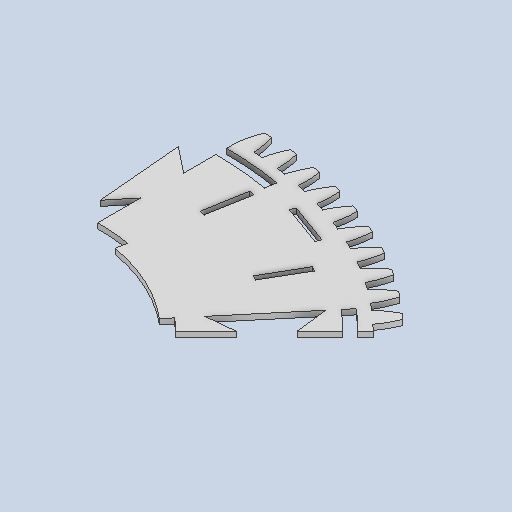
# Autodesk Inventor part: Base Plate Bottom v3
Saved by Autodesk Inventor 2023 (Build 270158000, 158)
## iProperties
Created: 2023-02-13
Part Number: Base Plate Bottom v3
Material: Generic
Document SubType Name: Sheet Metal
Designer: cheng
Density: 1 g/cm^3
Appearance: Default
Sheet Metal Rule: Default
Author: cheng
Autodesk Inventor part; units mm, degrees
(part 1 of 2)
ref_plane "YZ Plane" through (0, 0, 0) normal (1, 0, 0) x (0, 1, 0)
ref_plane "XZ Plane" through (0, 0, 0) normal (0, 1, 0) x (-1, 0, 0)
ref_plane "XY Plane" through (0, 0, 0) normal (0, 0, 1) x (1, 0, 0)
sketch "Sketch2" plane through (0, 0, 0) normal (0, 1, 0) x (-1, 0, 0)
  circle A0 centre (0, 0) radius 325
  circle A1 centre (0, 0) radius 165
  line L0 (0, 0) -> (0, -325)
  line L1 (0, 0) -> (-229.8097, -229.8097)
  line L2 (0, 0) -> (28.3256, -323.7633)
  line L3 (0, 0) -> (-208.906, -248.9644)
  circle A2 centre (0, 0) radius 275 construction
  circle A3 centre (0, 0) radius 195
  circle A4 centre (0, 0) radius 215
  circle A5 centre (0, 0) radius 255 construction
  line L4 (16.9954, -194.258) -> (0, -215)
  line L5 (23.9678, -273.9535) -> (0, -255)
  line L6 (-125.3436, -149.3787) -> (-152.028, -152.028)
  line L7 (-176.7666, -210.6622) -> (-180.3122, -180.3122)
  line L8 (0, 0) -> (-111.1565, -305.4001) construction
  circle A6 centre (0, 0) radius 235 construction
  circle A7 centre (0, 0) radius 275 construction
  line L9 (0, 0) -> (-17.0092, -324.5546) construction
  line L10 (0, 0) -> (-8.5075, -324.8886) construction
  circle A8 centre (0, 0) radius 305
  arc A9 (-5.1732, -324.9588) -> (0, -305) centre (-79.3819, -295.0744) ccw
  arc A10 (-15.9625, -304.582) -> (-11.8409, -324.7842) centre (63.8301, -298.8246) ccw
  arc A11 (20.3387, -324.363) -> (23.93, -304.0598) centre (-55.9859, -300.393) ccw
  arc A12 (7.984, -304.8955) -> (13.6779, -324.712) centre (87.0788, -292.8953) ccw
  arc A13 (45.7252, -321.7673) -> (47.7125, -301.2449) centre (-32.2447, -303.8596) ccw
  arc A14 (31.8812, -303.3292) -> (39.1123, -322.6379) centre (109.7907, -285.1603) ccw
  arc A15 (70.8298, -317.1879) -> (71.2008, -296.5728) centre (-8.3048, -305.4528) ccw
  arc A16 (55.5818, -299.8927) -> (64.3057, -318.5746) centre (131.8257, -275.6672) ccw
  arc A17 (95.4978, -310.6528) -> (94.2502, -290.0722) centre (15.6864, -305.1628) ccw
  arc A18 (78.9398, -294.6074) -> (89.1025, -312.5472) centre (153.0479, -264.4745) ccw
  arc A19 (119.5769, -302.2025) -> (116.7184, -281.7833) centre (39.5808, -302.9913) ccw
  arc A20 (101.8111, -287.5057) -> (113.35, -304.5928) centre (173.3265, -251.6512) ccw
  arc A21 (142.9188, -291.889) -> (138.4671, -271.757) centre (63.2312, -298.9518) ccw
  arc A22 (124.0547, -278.6314) -> (136.8987, -294.7605) centre (192.5365, -237.2764) ccw
  arc A23 (165.3796, -279.776) -> (159.3621, -260.0553) centre (86.4918, -293.0692) ccw
  arc A24 (145.5334, -268.0392) -> (159.6033, -283.1109) centre (210.5595, -221.4387) ccw
  arc A25 (186.8208, -265.938) -> (179.2745, -246.7502) centre (109.2191, -285.3797) ccw
  arc A26 (166.1149, -255.7945) -> (181.3239, -269.7159) centre (227.2843, -204.2358) ccw
  arc A27 (207.1101, -250.4604) -> (198.0817, -231.9238) centre (131.273, -275.9308) ccw
  arc A28 (185.6722, -241.9728) -> (201.9266, -254.6579) centre (242.6078, -185.7736) ccw
  arc A29 (226.1226, -233.4386) -> (215.6676, -215.6676) centre (152.5177, -264.7806) ccw
  arc A30 (204.0848, -226.6592) -> (221.2844, -238.0299) centre (256.4356, -166.1662) ccw
  arc A31 (243.7409, -214.9776) -> (231.9238, -198.0817) centre (172.8219, -251.998) ccw
  arc A32 (221.2392, -209.9481) -> (239.2778, -219.9344) centre (268.6823, -145.5342) ccw
  arc A33 (259.8565, -195.1912) -> (246.7502, -179.2745) centre (192.0607, -237.6617) ccw
  arc A34 (237.0295, -191.9427) -> (255.7961, -200.4829) centre (279.2725, -124.005) ccw
  arc A35 (274.3699, -174.2014) -> (260.0553, -159.3621) centre (210.1154, -221.8601) ccw
  arc A36 (251.3585, -172.7539) -> (270.7372, -179.7953) centre (288.1409, -101.7113) ccw
  arc A37 (287.1918, -152.1376) -> (271.757, -138.4671) centre (226.8746, -204.6908) ccw
  arc A38 (264.1377, -152.5) -> (284.0092, -157.9993) centre (295.2329, -78.7905) ccw
  arc A39 (298.2431, -129.1358) -> (281.7833, -116.7184) centre (242.2351, -186.2594) ccw
  arc A40 (275.2885, -131.3059) -> (295.5302, -135.2291) centre (300.5046, -55.3839) ccw
  arc A41 (307.4556, -105.3378) -> (290.0722, -94.2502) centre (256.1021, -166.6797) ccw
  arc A42 (284.742, -109.3022) -> (305.2291, -111.6252) centre (303.9236, -31.6358) ccw
  arc A43 (314.7725, -80.8904) -> (296.5728, -71.2008) centre (268.3902, -146.0723) ccw
  arc A44 (292.44, -86.6247) -> (313.0462, -87.3331) centre (305.4688, -7.6927) ccw
  arc A45 (320.1488, -55.9443) -> (301.2449, -47.7125) centre (279.0235, -124.5644) ccw
  arc A46 (298.335, -63.4131) -> (318.9333, -62.5025) centre (305.1308, 16.2978) ccw
  arc A47 (323.5512, -30.6533) -> (304.0598, -23.93) centre (287.9366, -102.2884) ccw
  arc A48 (302.3907, -39.8105) -> (322.854, -37.2867) centre (302.9114, 40.1878) ccw
  arc A49 (324.9588, -5.1732) -> (305, 0) centre (295.0744, -79.3819) ccw
  arc A50 (304.582, -15.9625) -> (324.7842, -11.8409) centre (298.8246, 63.8301) ccw
  arc A51 (324.363, 20.3387) -> (304.0598, 23.93) centre (300.393, -55.9859) ccw
  arc A52 (304.8955, 7.984) -> (324.712, 13.6779) centre (292.8953, 87.0788) ccw
  arc A53 (321.7673, 45.7252) -> (301.2449, 47.7125) centre (303.8596, -32.2447) ccw
  arc A54 (303.3292, 31.8812) -> (322.6379, 39.1123) centre (285.1603, 109.7907) ccw
  arc A55 (317.1879, 70.8298) -> (296.5728, 71.2008) centre (305.4528, -8.3048) ccw
  arc A56 (299.8927, 55.5818) -> (318.5746, 64.3057) centre (275.6672, 131.8257) ccw
  arc A57 (310.6528, 95.4978) -> (290.0722, 94.2502) centre (305.1628, 15.6864) ccw
  arc A58 (294.6074, 78.9398) -> (312.5472, 89.1025) centre (264.4745, 153.0479) ccw
  arc A59 (302.2025, 119.5769) -> (281.7833, 116.7184) centre (302.9913, 39.5808) ccw
  arc A60 (287.5057, 101.8111) -> (304.5928, 113.35) centre (251.6512, 173.3265) ccw
  arc A61 (291.889, 142.9188) -> (271.757, 138.4671) centre (298.9518, 63.2312) ccw
  arc A62 (278.6314, 124.0547) -> (294.7605, 136.8987) centre (237.2764, 192.5365) ccw
  arc A63 (279.776, 165.3796) -> (260.0553, 159.3621) centre (293.0692, 86.4918) ccw
  arc A64 (268.0392, 145.5334) -> (283.1109, 159.6033) centre (221.4387, 210.5595) ccw
  arc A65 (265.938, 186.8208) -> (246.7502, 179.2745) centre (285.3797, 109.2191) ccw
  arc A66 (255.7945, 166.1149) -> (269.7159, 181.3239) centre (204.2358, 227.2843) ccw
  arc A67 (250.4604, 207.1101) -> (231.9238, 198.0817) centre (275.9308, 131.273) ccw
  arc A68 (241.9728, 185.6722) -> (254.6579, 201.9266) centre (185.7736, 242.6078) ccw
  arc A69 (233.4386, 226.1226) -> (215.6676, 215.6676) centre (264.7806, 152.5177) ccw
  arc A70 (226.6592, 204.0848) -> (238.0299, 221.2844) centre (166.1662, 256.4356) ccw
  arc A71 (214.9776, 243.7409) -> (198.0817, 231.9238) centre (251.998, 172.8219) ccw
  arc A72 (209.9481, 221.2392) -> (219.9344, 239.2778) centre (145.5342, 268.6823) ccw
  arc A73 (195.1912, 259.8565) -> (179.2745, 246.7502) centre (237.6617, 192.0607) ccw
  arc A74 (191.9427, 237.0295) -> (200.4829, 255.7961) centre (124.005, 279.2725) ccw
  arc A75 (174.2014, 274.3699) -> (159.3621, 260.0553) centre (221.8601, 210.1154) ccw
  arc A76 (172.7539, 251.3585) -> (179.7953, 270.7372) centre (101.7113, 288.1409) ccw
  arc A77 (152.1376, 287.1918) -> (138.4671, 271.757) centre (204.6908, 226.8746) ccw
  arc A78 (152.5, 264.1377) -> (157.9993, 284.0092) centre (78.7905, 295.2329) ccw
  arc A79 (129.1358, 298.2431) -> (116.7184, 281.7833) centre (186.2594, 242.2351) ccw
  arc A80 (131.3059, 275.2885) -> (135.2291, 295.5302) centre (55.3839, 300.5046) ccw
  arc A81 (105.3378, 307.4556) -> (94.2502, 290.0722) centre (166.6797, 256.1021) ccw
  arc A82 (109.3022, 284.742) -> (111.6252, 305.2291) centre (31.6358, 303.9236) ccw
  arc A83 (80.8904, 314.7725) -> (71.2008, 296.5728) centre (146.0723, 268.3902) ccw
  arc A84 (86.6247, 292.44) -> (87.3331, 313.0462) centre (7.6927, 305.4688) ccw
  arc A85 (55.9443, 320.1488) -> (47.7125, 301.2449) centre (124.5644, 279.0235) ccw
  arc A86 (63.4131, 298.335) -> (62.5025, 318.9333) centre (-16.2978, 305.1308) ccw
  arc A87 (30.6533, 323.5512) -> (23.93, 304.0598) centre (102.2884, 287.9366) ccw
  arc A88 (39.8105, 302.3907) -> (37.2867, 322.854) centre (-40.1878, 302.9114) ccw
  circle A89 centre (0, 0) radius 295
  circle A90 centre (0, 0) radius 285
  line L11 (0, 0) -> (-52.9627, -300.3664)
  line L12 (-80.392, -279.3513) -> (-117.9797, -265.6705)
  line L13 (-117.9797, -265.6705) -> (-116.2696, -260.972)
  line L14 (-116.2696, -260.972) -> (-78.6819, -274.6528)
  line L15 (-78.6819, -274.6528) -> (-80.392, -279.3513)
  line L16 (-80.392, -279.3513) -> (-116.2696, -260.972) construction
  line L17 (-117.9797, -265.6705) -> (-78.6819, -274.6528) construction
  line L18 (-98.3308, -270.1616) -> (-99.1858, -272.5109)
  circle A91 centre (0, 0) radius 175
  line L19 (-135.3349, -239.407) -> (-139.6651, -236.907)
  line L20 (-139.6651, -236.907) -> (-119.6651, -202.266)
  line L21 (-119.6651, -202.266) -> (-115.3349, -204.766)
  line L22 (-115.3349, -204.766) -> (-135.3349, -239.407)
  line L23 (-135.3349, -239.407) -> (-119.6651, -202.266) construction
  line L24 (-139.6651, -236.907) -> (-115.3349, -204.766) construction
  line L25 (-137.5, -238.157) -> (-117.5, -203.516) construction
  line L26 (-129.6651, -219.5865) -> (-125.3349, -222.0865) construction
  line L27 (-50.2153, -270.388) -> (-45.2912, -271.2563)
  line L28 (-45.2912, -271.2563) -> (-38.3453, -231.8639)
  line L29 (-38.3453, -231.8639) -> (-43.2693, -230.9957)
  line L30 (-43.2693, -230.9957) -> (-50.2153, -270.388)
  line L31 (-50.2153, -270.388) -> (-38.3453, -231.8639) construction
  line L32 (-45.2912, -271.2563) -> (-43.2693, -230.9957) construction
  line L33 (-47.7532, -270.8221) -> (-40.8073, -231.4298) construction
  arc A92 (5.1732, 324.9588) -> (0, 305) centre (79.3819, 295.0744) ccw
  arc A93 (15.9625, 304.582) -> (11.8409, 324.7842) centre (-63.8301, 298.8246) ccw
  arc A94 (-20.3387, 324.363) -> (-23.93, 304.0598) centre (55.9859, 300.393) ccw
  arc A95 (-7.984, 304.8955) -> (-13.6779, 324.712) centre (-87.0788, 292.8953) ccw
  arc A96 (-45.7252, 321.7673) -> (-47.7125, 301.2449) centre (32.2447, 303.8596) ccw
  arc A97 (-31.8812, 303.3292) -> (-39.1123, 322.6379) centre (-109.7907, 285.1603) ccw
  arc A98 (-70.8298, 317.1879) -> (-71.2008, 296.5728) centre (8.3048, 305.4528) ccw
  arc A99 (-55.5818, 299.8927) -> (-64.3057, 318.5746) centre (-131.8257, 275.6672) ccw
  arc A100 (-95.4978, 310.6528) -> (-94.2502, 290.0722) centre (-15.6864, 305.1628) ccw
  arc A101 (-78.9398, 294.6074) -> (-89.1025, 312.5472) centre (-153.0479, 264.4745) ccw
  arc A102 (-119.5769, 302.2025) -> (-116.7184, 281.7833) centre (-39.5808, 302.9913) ccw
  arc A103 (-101.8111, 287.5057) -> (-113.35, 304.5928) centre (-173.3265, 251.6512) ccw
  arc A104 (-142.9188, 291.889) -> (-138.4671, 271.757) centre (-63.2312, 298.9518) ccw
  arc A105 (-124.0547, 278.6314) -> (-136.8987, 294.7605) centre (-192.5365, 237.2764) ccw
  arc A106 (-165.3796, 279.776) -> (-159.3621, 260.0553) centre (-86.4918, 293.0692) ccw
  arc A107 (-145.5334, 268.0392) -> (-159.6033, 283.1109) centre (-210.5595, 221.4387) ccw
  arc A108 (-186.8208, 265.938) -> (-179.2745, 246.7502) centre (-109.2191, 285.3797) ccw
  arc A109 (-166.1149, 255.7945) -> (-181.3239, 269.7159) centre (-227.2843, 204.2358) ccw
  arc A110 (-207.1101, 250.4604) -> (-198.0817, 231.9238) centre (-131.273, 275.9308) ccw
  arc A111 (-185.6722, 241.9728) -> (-201.9266, 254.6579) centre (-242.6078, 185.7736) ccw
  arc A112 (-226.1226, 233.4386) -> (-215.6676, 215.6676) centre (-152.5177, 264.7806) ccw
  arc A113 (-204.0848, 226.6592) -> (-221.2844, 238.0299) centre (-256.4356, 166.1662) ccw
  arc A114 (-243.7409, 214.9776) -> (-231.9238, 198.0817) centre (-172.8219, 251.998) ccw
  arc A115 (-221.2392, 209.9481) -> (-239.2778, 219.9344) centre (-268.6823, 145.5342) ccw
  arc A116 (-259.8565, 195.1912) -> (-246.7502, 179.2745) centre (-192.0607, 237.6617) ccw
  arc A117 (-237.0295, 191.9427) -> (-255.7961, 200.4829) centre (-279.2725, 124.005) ccw
  arc A118 (-274.3699, 174.2014) -> (-260.0553, 159.3621) centre (-210.1154, 221.8601) ccw
  arc A119 (-251.3585, 172.7539) -> (-270.7372, 179.7953) centre (-288.1409, 101.7113) ccw
  arc A120 (-287.1918, 152.1376) -> (-271.757, 138.4671) centre (-226.8746, 204.6908) ccw
  arc A121 (-264.1377, 152.5) -> (-284.0092, 157.9993) centre (-295.2329, 78.7905) ccw
  arc A122 (-298.2431, 129.1358) -> (-281.7833, 116.7184) centre (-242.2351, 186.2594) ccw
  arc A123 (-275.2885, 131.3059) -> (-295.5302, 135.2291) centre (-300.5046, 55.3839) ccw
  arc A124 (-307.4556, 105.3378) -> (-290.0722, 94.2502) centre (-256.1021, 166.6797) ccw
  arc A125 (-284.742, 109.3022) -> (-305.2291, 111.6252) centre (-303.9236, 31.6358) ccw
  arc A126 (-314.7725, 80.8904) -> (-296.5728, 71.2008) centre (-268.3902, 146.0723) ccw
  arc A127 (-292.44, 86.6247) -> (-313.0462, 87.3331) centre (-305.4688, 7.6927) ccw
  arc A128 (-320.1488, 55.9443) -> (-301.2449, 47.7125) centre (-279.0235, 124.5644) ccw
  arc A129 (-298.335, 63.4131) -> (-318.9333, 62.5025) centre (-305.1308, -16.2978) ccw
  arc A130 (-323.5512, 30.6533) -> (-304.0598, 23.93) centre (-287.9366, 102.2884) ccw
  arc A131 (-302.3907, 39.8105) -> (-322.854, 37.2867) centre (-302.9114, -40.1878) ccw
  arc A132 (-324.9588, 5.1732) -> (-305, 0) centre (-295.0744, 79.3819) ccw
  arc A133 (-304.582, 15.9625) -> (-324.7842, 11.8409) centre (-298.8246, -63.8301) ccw
  arc A134 (-324.363, -20.3387) -> (-304.0598, -23.93) centre (-300.393, 55.9859) ccw
  arc A135 (-304.8955, -7.984) -> (-324.712, -13.6779) centre (-292.8953, -87.0788) ccw
  arc A136 (-321.7673, -45.7252) -> (-301.2449, -47.7125) centre (-303.8596, 32.2447) ccw
  arc A137 (-303.3292, -31.8812) -> (-322.6379, -39.1123) centre (-285.1603, -109.7907) ccw
  arc A138 (-317.1879, -70.8298) -> (-296.5728, -71.2008) centre (-305.4528, 8.3048) ccw
  arc A139 (-299.8927, -55.5818) -> (-318.5746, -64.3057) centre (-275.6672, -131.8257) ccw
  arc A140 (-310.6528, -95.4978) -> (-290.0722, -94.2502) centre (-305.1628, -15.6864) ccw
  arc A141 (-294.6074, -78.9398) -> (-312.5472, -89.1025) centre (-264.4745, -153.0479) ccw
  arc A142 (-302.2025, -119.5769) -> (-281.7833, -116.7184) centre (-302.9913, -39.5808) ccw
  arc A143 (-287.5057, -101.8111) -> (-304.5928, -113.35) centre (-251.6512, -173.3265) ccw
  arc A144 (-291.889, -142.9188) -> (-271.757, -138.4671) centre (-298.9518, -63.2312) ccw
  arc A145 (-278.6314, -124.0547) -> (-294.7605, -136.8987) centre (-237.2764, -192.5365) ccw
  arc A146 (-279.776, -165.3796) -> (-260.0553, -159.3621) centre (-293.0692, -86.4918) ccw
  arc A147 (-268.0392, -145.5334) -> (-283.1109, -159.6033) centre (-221.4387, -210.5595) ccw
  arc A148 (-265.938, -186.8208) -> (-246.7502, -179.2745) centre (-285.3797, -109.2191) ccw
  arc A149 (-255.7945, -166.1149) -> (-269.7159, -181.3239) centre (-204.2358, -227.2843) ccw
  arc A150 (-250.4604, -207.1101) -> (-231.9238, -198.0817) centre (-275.9308, -131.273) ccw
  arc A151 (-241.9728, -185.6722) -> (-254.6579, -201.9266) centre (-185.7736, -242.6078) ccw
  arc A152 (-233.4386, -226.1226) -> (-215.6676, -215.6676) centre (-264.7806, -152.5177) ccw
  arc A153 (-226.6592, -204.0848) -> (-238.0299, -221.2844) centre (-166.1662, -256.4356) ccw
  arc A154 (-214.9776, -243.7409) -> (-198.0817, -231.9238) centre (-251.998, -172.8219) ccw
  arc A155 (-209.9481, -221.2392) -> (-219.9344, -239.2778) centre (-145.5342, -268.6823) ccw
  arc A156 (-195.1912, -259.8565) -> (-179.2745, -246.7502) centre (-237.6617, -192.0607) ccw
  arc A157 (-191.9427, -237.0295) -> (-200.4829, -255.7961) centre (-124.005, -279.2725) ccw
  arc A158 (-174.2014, -274.3699) -> (-159.3621, -260.0553) centre (-221.8601, -210.1154) ccw
  arc A159 (-172.7539, -251.3585) -> (-179.7953, -270.7372) centre (-101.7113, -288.1409) ccw
  arc A160 (-152.1376, -287.1918) -> (-138.4671, -271.757) centre (-204.6908, -226.8746) ccw
  arc A161 (-152.5, -264.1377) -> (-157.9993, -284.0092) centre (-78.7905, -295.2329) ccw
  arc A162 (-129.1358, -298.2431) -> (-116.7184, -281.7833) centre (-186.2594, -242.2351) ccw
  arc A163 (-131.3059, -275.2885) -> (-135.2291, -295.5302) centre (-55.3839, -300.5046) ccw
  arc A164 (-105.3378, -307.4556) -> (-94.2502, -290.0722) centre (-166.6797, -256.1021) ccw
  arc A165 (-109.3022, -284.742) -> (-111.6252, -305.2291) centre (-31.6358, -303.9236) ccw
  arc A166 (-80.8904, -314.7725) -> (-71.2008, -296.5728) centre (-146.0723, -268.3902) ccw
  arc A167 (-86.6247, -292.44) -> (-87.3331, -313.0462) centre (-7.6927, -305.4688) ccw
  arc A168 (-55.9443, -320.1488) -> (-47.7125, -301.2449) centre (-124.5644, -279.0235) ccw
  arc A169 (-63.4131, -298.335) -> (-62.5025, -318.9333) centre (16.2978, -305.1308) ccw
  arc A170 (-30.6533, -323.5512) -> (-23.93, -304.0598) centre (-102.2884, -287.9366) ccw
  arc A171 (-39.8105, -302.3907) -> (-37.2867, -322.854) centre (40.1878, -302.9114) ccw
  line L34 (155.6856, -226.7008) -> (159.7814, -223.8329)
  line L35 (159.7814, -223.8329) -> (132.7426, -193.9347) construction
  line L36 (132.7426, -193.9347) -> (155.6856, -226.7008)
  line L37 (157.7335, -225.2668) -> (134.7905, -192.5007) construction
  line L38 (155.6856, -226.7008) -> (136.8383, -191.0668) construction
  line L39 (159.7814, -223.8329) -> (136.8383, -191.0668)
  line L40 (136.8383, -191.0668) -> (132.7426, -193.9347)
  line L41 (149.3787, -125.3436) -> (152.028, -152.028)
  line L42 (210.6622, -176.7666) -> (180.3122, -180.3122)
  arc A172 (243.7409, -214.9776) -> (231.9238, -198.0817) centre (172.8219, -251.998) ccw
  arc A173 (221.2392, -209.9481) -> (239.2778, -219.9344) centre (268.6823, -145.5342) ccw
  arc A174 (259.8565, -195.1912) -> (246.7502, -179.2745) centre (192.0607, -237.6617) ccw
  arc A175 (237.0295, -191.9427) -> (255.7961, -200.4829) centre (279.2725, -124.005) ccw
  line L43 (16.9954, -194.258) -> (0, -215)
  line L44 (63.584, -246.9581) -> (68.4137, -245.664) construction
  line L45 (63.2373, -226.3455) -> (73.5901, -264.9826)
  arc A176 (226.1226, -233.4386) -> (215.6676, -215.6676) centre (152.5177, -264.7806) ccw
  arc A177 (204.0848, -226.6592) -> (221.2844, -238.0299) centre (256.4356, -166.1662) ccw
  arc A178 (185.6722, -241.9728) -> (201.9266, -254.6579) centre (242.6078, -185.7736) ccw
  arc A179 (207.1101, -250.4604) -> (198.0817, -231.9238) centre (131.273, -275.9308) ccw
  line L46 (138.5724, -249.8454) -> (140.6855, -254.3769)
  arc A180 (186.8208, -265.938) -> (179.2745, -246.7502) centre (109.2191, -285.3797) ccw
  arc A181 (166.1149, -255.7945) -> (181.3239, -269.7159) centre (227.2843, -204.2358) ccw
  arc A182 (165.3796, -279.776) -> (159.3621, -260.0553) centre (86.4918, -293.0692) ccw
  arc A183 (145.5334, -268.0392) -> (159.6033, -283.1109) centre (210.5595, -221.4387) ccw
  line L47 (140.6855, -254.3769) -> (104.4331, -271.2816)
  line L48 (102.32, -266.7501) -> (138.5724, -249.8454)
  line L49 (140.6855, -254.3769) -> (102.32, -266.7501) construction
  line L50 (104.4331, -271.2816) -> (138.5724, -249.8454) construction
  arc A184 (101.8111, -287.5057) -> (113.35, -304.5928) centre (173.3265, -251.6512) ccw
  arc A185 (119.5769, -302.2025) -> (116.7184, -281.7833) centre (39.5808, -302.9913) ccw
  arc A186 (124.0547, -278.6314) -> (136.8987, -294.7605) centre (192.5365, -237.2764) ccw
  arc A187 (142.9188, -291.889) -> (138.4671, -271.757) centre (63.2312, -298.9518) ccw
  arc A188 (95.4978, -310.6528) -> (94.2502, -290.0722) centre (15.6864, -305.1628) ccw
  line L51 (104.4331, -271.2816) -> (102.32, -266.7501)
  line L52 (121.5028, -260.5635) -> (122.5593, -262.8293)
  arc A189 (70.8298, -317.1879) -> (71.2008, -296.5728) centre (-8.3048, -305.4528) ccw
  arc A190 (55.5818, -299.8927) -> (64.3057, -318.5746) centre (131.8257, -275.6672) ccw
  arc A191 (78.9398, -294.6074) -> (89.1025, -312.5472) centre (153.0479, -264.4745) ccw
  line L53 (23.9678, -273.9535) -> (0, -255)
  arc A192 (-5.1732, -324.9588) -> (0, -305) centre (-79.3819, -295.0744) ccw
  arc A193 (7.984, -304.8955) -> (13.6779, -324.712) centre (87.0788, -292.8953) ccw
  arc A194 (20.3387, -324.363) -> (23.93, -304.0598) centre (-55.9859, -300.393) ccw
  arc A195 (31.8812, -303.3292) -> (39.1123, -322.6379) centre (109.7907, -285.1603) ccw
  arc A196 (45.7252, -321.7673) -> (47.7125, -301.2449) centre (-32.2447, -303.8596) ccw
  line L54 (73.5901, -264.9826) -> (68.7604, -266.2766)
  line L55 (0, 0) -> (229.8097, -229.8097)
  line L56 (0, 0) -> (0, -325)
  line L57 (0, 0) -> (248.9644, -208.906)
  line L58 (0, 0) -> (28.3256, -323.7633)
  line L59 (58.4077, -227.6396) -> (63.2373, -226.3455)
  line L60 (71.1752, -265.6296) -> (60.8225, -226.9926) construction
  line L61 (68.7604, -266.2766) -> (63.2373, -226.3455) construction
  line L62 (68.7604, -266.2766) -> (58.4077, -227.6396)
  line L63 (73.5901, -264.9826) -> (58.4077, -227.6396) construction
  line L64 (0, 0) -> (223.7152, -235.7467) construction
  line L65 (0, 0) -> (217.4674, -241.5221) construction
  line L66 (0, 0) -> (174.9408, -249.8414)
  line L67 (0, 0) -> (137.3509, -294.55) construction
  line L68 (270.388, -50.2153) -> (271.2563, -45.2912)
  line L69 (271.2563, -45.2912) -> (230.9957, -43.2693) construction
  line L70 (230.9957, -43.2693) -> (270.388, -50.2153)
  line L71 (270.8221, -47.7532) -> (231.4298, -40.8073) construction
  line L72 (270.388, -50.2153) -> (231.8639, -38.3453) construction
  line L73 (271.2563, -45.2912) -> (231.8639, -38.3453)
  line L74 (231.8639, -38.3453) -> (230.9957, -43.2693)
  line L75 (194.258, 16.9954) -> (215, 0)
  line L76 (273.9535, 23.9678) -> (255, 0)
  arc A197 (324.363, 20.3387) -> (304.0598, 23.93) centre (300.393, -55.9859) ccw
  arc A198 (304.8955, 7.984) -> (324.712, 13.6779) centre (292.8953, 87.0788) ccw
  arc A199 (321.7673, 45.7252) -> (301.2449, 47.7125) centre (303.8596, -32.2447) ccw
  arc A200 (303.3292, 31.8812) -> (322.6379, 39.1123) centre (285.1603, 109.7907) ccw
  line L77 (149.3787, -125.3436) -> (152.028, -152.028)
  line L78 (219.5865, -129.6651) -> (222.0865, -125.3349) construction
  line L79 (204.766, -115.3349) -> (239.407, -135.3349)
  arc A201 (324.9588, -5.1732) -> (305, 0) centre (295.0744, -79.3819) ccw
  arc A202 (304.582, -15.9625) -> (324.7842, -11.8409) centre (298.8246, 63.8301) ccw
  arc A203 (302.3907, -39.8105) -> (322.854, -37.2867) centre (302.9114, 40.1878) ccw
  arc A204 (323.5512, -30.6533) -> (304.0598, -23.93) centre (287.9366, -102.2884) ccw
  line L80 (274.6528, -78.6819) -> (279.3513, -80.392)
  arc A205 (320.1488, -55.9443) -> (301.2449, -47.7125) centre (279.0235, -124.5644) ccw
  arc A206 (298.335, -63.4131) -> (318.9333, -62.5025) centre (305.1308, 16.2978) ccw
  arc A207 (314.7725, -80.8904) -> (296.5728, -71.2008) centre (268.3902, -146.0723) ccw
  arc A208 (292.44, -86.6247) -> (313.0462, -87.3331) centre (305.4688, -7.6927) ccw
  line L81 (279.3513, -80.392) -> (265.6705, -117.9797)
  line L82 (260.972, -116.2696) -> (274.6528, -78.6819)
  line L83 (279.3513, -80.392) -> (260.972, -116.2696) construction
  line L84 (265.6705, -117.9797) -> (274.6528, -78.6819) construction
  arc A209 (275.2885, -131.3059) -> (295.5302, -135.2291) centre (300.5046, -55.3839) ccw
  arc A210 (298.2431, -129.1358) -> (281.7833, -116.7184) centre (242.2351, -186.2594) ccw
  arc A211 (284.742, -109.3022) -> (305.2291, -111.6252) centre (303.9236, -31.6358) ccw
  arc A212 (307.4556, -105.3378) -> (290.0722, -94.2502) centre (256.1021, -166.6797) ccw
  arc A213 (287.1918, -152.1376) -> (271.757, -138.4671) centre (226.8746, -204.6908) ccw
  line L85 (265.6705, -117.9797) -> (260.972, -116.2696)
  line L86 (270.1616, -98.3308) -> (272.5109, -99.1858)
  arc A214 (274.3699, -174.2014) -> (260.0553, -159.3621) centre (210.1154, -221.8601) ccw
  arc A215 (251.3585, -172.7539) -> (270.7372, -179.7953) centre (288.1409, -101.7113) ccw
  arc A216 (264.1377, -152.5) -> (284.0092, -157.9993) centre (295.2329, -78.7905) ccw
  line L87 (210.6622, -176.7666) -> (180.3122, -180.3122)
  arc A217 (226.1226, -233.4386) -> (215.6676, -215.6676) centre (152.5177, -264.7806) ccw
  arc A218 (221.2392, -209.9481) -> (239.2778, -219.9344) centre (268.6823, -145.5342) ccw
  arc A219 (243.7409, -214.9776) -> (231.9238, -198.0817) centre (172.8219, -251.998) ccw
  arc A220 (237.0295, -191.9427) -> (255.7961, -200.4829) centre (279.2725, -124.005) ccw
  arc A221 (259.8565, -195.1912) -> (246.7502, -179.2745) centre (192.0607, -237.6617) ccw
  line L88 (239.407, -135.3349) -> (236.907, -139.6651)
  line L89 (0, 0) -> (325, 0)
  line L90 (0, 0) -> (229.8097, -229.8097)
  line L91 (0, 0) -> (323.7633, 28.3256)
  line L92 (0, 0) -> (248.9644, -208.906)
  line L93 (202.266, -119.6651) -> (204.766, -115.3349)
  line L94 (238.157, -137.5) -> (203.516, -117.5) construction
  line L95 (236.907, -139.6651) -> (204.766, -115.3349) construction
  line L96 (236.907, -139.6651) -> (202.266, -119.6651)
  line L97 (239.407, -135.3349) -> (202.266, -119.6651) construction
  line L98 (0, 0) -> (324.8886, -8.5075) construction
  line L99 (0, 0) -> (324.5546, -17.0092) construction
  line L100 (0, 0) -> (300.3664, -52.9627)
  line L101 (0, 0) -> (305.4001, -111.1565) construction
  line L102 (226.7008, 155.6856) -> (223.8329, 159.7814)
  line L103 (223.8329, 159.7814) -> (193.9347, 132.7426) construction
  line L104 (193.9347, 132.7426) -> (226.7008, 155.6856)
  line L105 (225.2668, 157.7335) -> (192.5007, 134.7905) construction
  line L106 (226.7008, 155.6856) -> (191.0668, 136.8383) construction
  line L107 (223.8329, 159.7814) -> (191.0668, 136.8383)
  line L108 (191.0668, 136.8383) -> (193.9347, 132.7426)
  line L109 (125.3436, 149.3787) -> (152.028, 152.028)
  line L110 (176.7666, 210.6622) -> (180.3122, 180.3122)
  arc A222 (214.9776, 243.7409) -> (198.0817, 231.9238) centre (251.998, 172.8219) ccw
  arc A223 (209.9481, 221.2392) -> (219.9344, 239.2778) centre (145.5342, 268.6823) ccw
  arc A224 (195.1912, 259.8565) -> (179.2745, 246.7502) centre (237.6617, 192.0607) ccw
  arc A225 (191.9427, 237.0295) -> (200.4829, 255.7961) centre (124.005, 279.2725) ccw
  line L111 (194.258, 16.9954) -> (215, 0)
  line L112 (246.9581, 63.584) -> (245.664, 68.4137) construction
  line L113 (226.3455, 63.2373) -> (264.9826, 73.5901)
  arc A226 (233.4386, 226.1226) -> (215.6676, 215.6676) centre (264.7806, 152.5177) ccw
  arc A227 (226.6592, 204.0848) -> (238.0299, 221.2844) centre (166.1662, 256.4356) ccw
  arc A228 (241.9728, 185.6722) -> (254.6579, 201.9266) centre (185.7736, 242.6078) ccw
  arc A229 (250.4604, 207.1101) -> (231.9238, 198.0817) centre (275.9308, 131.273) ccw
  line L114 (249.8454, 138.5724) -> (254.3769, 140.6855)
  arc A230 (265.938, 186.8208) -> (246.7502, 179.2745) centre (285.3797, 109.2191) ccw
  arc A231 (255.7945, 166.1149) -> (269.7159, 181.3239) centre (204.2358, 227.2843) ccw
  arc A232 (279.776, 165.3796) -> (260.0553, 159.3621) centre (293.0692, 86.4918) ccw
  arc A233 (268.0392, 145.5334) -> (283.1109, 159.6033) centre (221.4387, 210.5595) ccw
  line L115 (254.3769, 140.6855) -> (271.2816, 104.4331)
  line L116 (266.7501, 102.32) -> (249.8454, 138.5724)
  line L117 (254.3769, 140.6855) -> (266.7501, 102.32) construction
  line L118 (271.2816, 104.4331) -> (249.8454, 138.5724) construction
  arc A234 (287.5057, 101.8111) -> (304.5928, 113.35) centre (251.6512, 173.3265) ccw
  arc A235 (302.2025, 119.5769) -> (281.7833, 116.7184) centre (302.9913, 39.5808) ccw
  arc A236 (278.6314, 124.0547) -> (294.7605, 136.8987) centre (237.2764, 192.5365) ccw
  arc A237 (291.889, 142.9188) -> (271.757, 138.4671) centre (298.9518, 63.2312) ccw
  arc A238 (310.6528, 95.4978) -> (290.0722, 94.2502) centre (305.1628, 15.6864) ccw
  line L119 (271.2816, 104.4331) -> (266.7501, 102.32)
  line L120 (260.5635, 121.5028) -> (262.8293, 122.5593)
  arc A239 (317.1879, 70.8298) -> (296.5728, 71.2008) centre (305.4528, -8.3048) ccw
  arc A240 (299.8927, 55.5818) -> (318.5746, 64.3057) centre (275.6672, 131.8257) ccw
  arc A241 (294.6074, 78.9398) -> (312.5472, 89.1025) centre (264.4745, 153.0479) ccw
  line L121 (273.9535, 23.9678) -> (255, 0)
  arc A242 (324.9588, -5.1732) -> (305, 0) centre (295.0744, -79.3819) ccw
  arc A243 (304.8955, 7.984) -> (324.712, 13.6779) centre (292.8953, 87.0788) ccw
  arc A244 (324.363, 20.3387) -> (304.0598, 23.93) centre (300.393, -55.9859) ccw
  arc A245 (303.3292, 31.8812) -> (322.6379, 39.1123) centre (285.1603, 109.7907) ccw
  arc A246 (321.7673, 45.7252) -> (301.2449, 47.7125) centre (303.8596, -32.2447) ccw
  line L122 (264.9826, 73.5901) -> (266.2766, 68.7604)
  line L123 (0, 0) -> (229.8097, 229.8097)
  line L124 (0, 0) -> (325, 0)
  line L125 (0, 0) -> (208.906, 248.9644)
  line L126 (0, 0) -> (323.7633, 28.3256)
  line L127 (227.6396, 58.4077) -> (226.3455, 63.2373)
  line L128 (265.6296, 71.1752) -> (226.9926, 60.8225) construction
  line L129 (266.2766, 68.7604) -> (226.3455, 63.2373) construction
  line L130 (266.2766, 68.7604) -> (227.6396, 58.4077)
  line L131 (264.9826, 73.5901) -> (227.6396, 58.4077) construction
  line L132 (0, 0) -> (235.7467, 223.7152) construction
  line L133 (0, 0) -> (241.5221, 217.4674) construction
  line L134 (0, 0) -> (249.8414, 174.9408)
  line L135 (0, 0) -> (294.55, 137.3509) construction
  line L136 (50.2153, 270.388) -> (45.2912, 271.2563)
  line L137 (45.2912, 271.2563) -> (43.2693, 230.9957) construction
  line L138 (43.2693, 230.9957) -> (50.2153, 270.388)
  line L139 (47.7532, 270.8221) -> (40.8073, 231.4298) construction
  line L140 (50.2153, 270.388) -> (38.3453, 231.8639) construction
  line L141 (45.2912, 271.2563) -> (38.3453, 231.8639)
  line L142 (38.3453, 231.8639) -> (43.2693, 230.9957)
  line L143 (-16.9954, 194.258) -> (0, 215)
  line L144 (-23.9678, 273.9535) -> (0, 255)
  arc A247 (-20.3387, 324.363) -> (-23.93, 304.0598) centre (55.9859, 300.393) ccw
  arc A248 (-7.984, 304.8955) -> (-13.6779, 324.712) centre (-87.0788, 292.8953) ccw
  arc A249 (-45.7252, 321.7673) -> (-47.7125, 301.2449) centre (32.2447, 303.8596) ccw
  arc A250 (-31.8812, 303.3292) -> (-39.1123, 322.6379) centre (-109.7907, 285.1603) ccw
  line L145 (125.3436, 149.3787) -> (152.028, 152.028)
  line L146 (129.6651, 219.5865) -> (125.3349, 222.0865) construction
  line L147 (115.3349, 204.766) -> (135.3349, 239.407)
  arc A251 (5.1732, 324.9588) -> (0, 305) centre (79.3819, 295.0744) ccw
  arc A252 (15.9625, 304.582) -> (11.8409, 324.7842) centre (-63.8301, 298.8246) ccw
  arc A253 (39.8105, 302.3907) -> (37.2867, 322.854) centre (-40.1878, 302.9114) ccw
  arc A254 (30.6533, 323.5512) -> (23.93, 304.0598) centre (102.2884, 287.9366) ccw
  line L148 (78.6819, 274.6528) -> (80.392, 279.3513)
  arc A255 (55.9443, 320.1488) -> (47.7125, 301.2449) centre (124.5644, 279.0235) ccw
  arc A256 (63.4131, 298.335) -> (62.5025, 318.9333) centre (-16.2978, 305.1308) ccw
  arc A257 (80.8904, 314.7725) -> (71.2008, 296.5728) centre (146.0723, 268.3902) ccw
  arc A258 (86.6247, 292.44) -> (87.3331, 313.0462) centre (7.6927, 305.4688) ccw
  line L149 (80.392, 279.3513) -> (117.9797, 265.6705)
  line L150 (116.2696, 260.972) -> (78.6819, 274.6528)
  line L151 (80.392, 279.3513) -> (116.2696, 260.972) construction
  line L152 (117.9797, 265.6705) -> (78.6819, 274.6528) construction
  arc A259 (131.3059, 275.2885) -> (135.2291, 295.5302) centre (55.3839, 300.5046) ccw
  arc A260 (129.1358, 298.2431) -> (116.7184, 281.7833) centre (186.2594, 242.2351) ccw
  arc A261 (109.3022, 284.742) -> (111.6252, 305.2291) centre (31.6358, 303.9236) ccw
  arc A262 (105.3378, 307.4556) -> (94.2502, 290.0722) centre (166.6797, 256.1021) ccw
  arc A263 (152.1376, 287.1918) -> (138.4671, 271.757) centre (204.6908, 226.8746) ccw
  line L153 (117.9797, 265.6705) -> (116.2696, 260.972)
  line L154 (98.3308, 270.1616) -> (99.1858, 272.5109)
  arc A264 (174.2014, 274.3699) -> (159.3621, 260.0553) centre (221.8601, 210.1154) ccw
  arc A265 (172.7539, 251.3585) -> (179.7953, 270.7372) centre (101.7113, 288.1409) ccw
  arc A266 (152.5, 264.1377) -> (157.9993, 284.0092) centre (78.7905, 295.2329) ccw
  line L155 (176.7666, 210.6622) -> (180.3122, 180.3122)
  arc A267 (233.4386, 226.1226) -> (215.6676, 215.6676) centre (264.7806, 152.5177) ccw
  arc A268 (209.9481, 221.2392) -> (219.9344, 239.2778) centre (145.5342, 268.6823) ccw
  arc A269 (214.9776, 243.7409) -> (198.0817, 231.9238) centre (251.998, 172.8219) ccw
  arc A270 (191.9427, 237.0295) -> (200.4829, 255.7961) centre (124.005, 279.2725) ccw
  arc A271 (195.1912, 259.8565) -> (179.2745, 246.7502) centre (237.6617, 192.0607) ccw
  line L156 (135.3349, 239.407) -> (139.6651, 236.907)
  line L157 (0, 0) -> (0, 325)
  line L158 (0, 0) -> (229.8097, 229.8097)
  line L159 (0, 0) -> (-28.3256, 323.7633)
  line L160 (0, 0) -> (208.906, 248.9644)
  line L161 (119.6651, 202.266) -> (115.3349, 204.766)
  line L162 (137.5, 238.157) -> (117.5, 203.516) construction
  line L163 (139.6651, 236.907) -> (115.3349, 204.766) construction
  line L164 (139.6651, 236.907) -> (119.6651, 202.266)
  line L165 (135.3349, 239.407) -> (119.6651, 202.266) construction
  line L166 (0, 0) -> (8.5075, 324.8886) construction
  line L167 (0, 0) -> (17.0092, 324.5546) construction
  line L168 (0, 0) -> (52.9627, 300.3664)
  line L169 (0, 0) -> (111.1565, 305.4001) construction
  line L170 (-155.6856, 226.7008) -> (-159.7814, 223.8329)
  line L171 (-159.7814, 223.8329) -> (-132.7426, 193.9347) construction
  line L172 (-132.7426, 193.9347) -> (-155.6856, 226.7008)
  line L173 (-157.7335, 225.2668) -> (-134.7905, 192.5007) construction
  line L174 (-155.6856, 226.7008) -> (-136.8383, 191.0668) construction
  line L175 (-159.7814, 223.8329) -> (-136.8383, 191.0668)
  line L176 (-136.8383, 191.0668) -> (-132.7426, 193.9347)
  line L177 (-149.3787, 125.3436) -> (-152.028, 152.028)
  line L178 (-210.6622, 176.7666) -> (-180.3122, 180.3122)
  arc A272 (-243.7409, 214.9776) -> (-231.9238, 198.0817) centre (-172.8219, 251.998) ccw
  arc A273 (-221.2392, 209.9481) -> (-239.2778, 219.9344) centre (-268.6823, 145.5342) ccw
  arc A274 (-259.8565, 195.1912) -> (-246.7502, 179.2745) centre (-192.0607, 237.6617) ccw
  arc A275 (-237.0295, 191.9427) -> (-255.7961, 200.4829) centre (-279.2725, 124.005) ccw
  line L179 (-16.9954, 194.258) -> (0, 215)
  line L180 (-63.584, 246.9581) -> (-68.4137, 245.664) construction
  line L181 (-63.2373, 226.3455) -> (-73.5901, 264.9826)
  arc A276 (-226.1226, 233.4386) -> (-215.6676, 215.6676) centre (-152.5177, 264.7806) ccw
  arc A277 (-204.0848, 226.6592) -> (-221.2844, 238.0299) centre (-256.4356, 166.1662) ccw
  arc A278 (-185.6722, 241.9728) -> (-201.9266, 254.6579) centre (-242.6078, 185.7736) ccw
  arc A279 (-207.1101, 250.4604) -> (-198.0817, 231.9238) centre (-131.273, 275.9308) ccw
  line L182 (-138.5724, 249.8454) -> (-140.6855, 254.3769)
  arc A280 (-186.8208, 265.938) -> (-179.2745, 246.7502) centre (-109.2191, 285.3797) ccw
  arc A281 (-166.1149, 255.7945) -> (-181.3239, 269.7159) centre (-227.2843, 204.2358) ccw
  arc A282 (-165.3796, 279.776) -> (-159.3621, 260.0553) centre (-86.4918, 293.0692) ccw
  arc A283 (-145.5334, 268.0392) -> (-159.6033, 283.1109) centre (-210.5595, 221.4387) ccw
  line L183 (-140.6855, 254.3769) -> (-104.4331, 271.2816)
  line L184 (-102.32, 266.7501) -> (-138.5724, 249.8454)
  line L185 (-140.6855, 254.3769) -> (-102.32, 266.7501) construction
  line L186 (-104.4331, 271.2816) -> (-138.5724, 249.8454) construction
  arc A284 (-101.8111, 287.5057) -> (-113.35, 304.5928) centre (-173.3265, 251.6512) ccw
  arc A285 (-119.5769, 302.2025) -> (-116.7184, 281.7833) centre (-39.5808, 302.9913) ccw
  arc A286 (-124.0547, 278.6314) -> (-136.8987, 294.7605) centre (-192.5365, 237.2764) ccw
  arc A287 (-142.9188, 291.889) -> (-138.4671, 271.757) centre (-63.2312, 298.9518) ccw
  arc A288 (-95.4978, 310.6528) -> (-94.2502, 290.0722) centre (-15.6864, 305.1628) ccw
  line L187 (-104.4331, 271.2816) -> (-102.32, 266.7501)
  line L188 (-121.5028, 260.5635) -> (-122.5593, 262.8293)
  arc A289 (-70.8298, 317.1879) -> (-71.2008, 296.5728) centre (8.3048, 305.4528) ccw
  arc A290 (-55.5818, 299.8927) -> (-64.3057, 318.5746) centre (-131.8257, 275.6672) ccw
  arc A291 (-78.9398, 294.6074) -> (-89.1025, 312.5472) centre (-153.0479, 264.4745) ccw
  line L189 (-23.9678, 273.9535) -> (0, 255)
  arc A292 (5.1732, 324.9588) -> (0, 305) centre (79.3819, 295.0744) ccw
  arc A293 (-7.984, 304.8955) -> (-13.6779, 324.712) centre (-87.0788, 292.8953) ccw
  arc A294 (-20.3387, 324.363) -> (-23.93, 304.0598) centre (55.9859, 300.393) ccw
  arc A295 (-31.8812, 303.3292) -> (-39.1123, 322.6379) centre (-109.7907, 285.1603) ccw
  arc A296 (-45.7252, 321.7673) -> (-47.7125, 301.2449) centre (32.2447, 303.8596) ccw
  line L190 (-73.5901, 264.9826) -> (-68.7604, 266.2766)
  line L191 (0, 0) -> (-229.8097, 229.8097)
  line L192 (0, 0) -> (0, 325)
  line L193 (0, 0) -> (-248.9644, 208.906)
  line L194 (0, 0) -> (-28.3256, 323.7633)
  line L195 (-58.4077, 227.6396) -> (-63.2373, 226.3455)
  line L196 (-71.1752, 265.6296) -> (-60.8225, 226.9926) construction
  line L197 (-68.7604, 266.2766) -> (-63.2373, 226.3455) construction
  line L198 (-68.7604, 266.2766) -> (-58.4077, 227.6396)
  line L199 (-73.5901, 264.9826) -> (-58.4077, 227.6396) construction
  line L200 (0, 0) -> (-223.7152, 235.7467) construction
  line L201 (0, 0) -> (-217.4674, 241.5221) construction
  line L202 (0, 0) -> (-174.9408, 249.8414)
  line L203 (0, 0) -> (-137.3509, 294.55) construction
  line L204 (-270.388, 50.2153) -> (-271.2563, 45.2912)
  line L205 (-271.2563, 45.2912) -> (-230.9957, 43.2693) construction
  line L206 (-230.9957, 43.2693) -> (-270.388, 50.2153)
  line L207 (-270.8221, 47.7532) -> (-231.4298, 40.8073) construction
  line L208 (-270.388, 50.2153) -> (-231.8639, 38.3453) construction
  line L209 (-271.2563, 45.2912) -> (-231.8639, 38.3453)
  line L210 (-231.8639, 38.3453) -> (-230.9957, 43.2693)
  line L211 (-194.258, -16.9954) -> (-215, 0)
  line L212 (-273.9535, -23.9678) -> (-255, 0)
  arc A297 (-324.363, -20.3387) -> (-304.0598, -23.93) centre (-300.393, 55.9859) ccw
  arc A298 (-304.8955, -7.984) -> (-324.712, -13.6779) centre (-292.8953, -87.0788) ccw
  arc A299 (-321.7673, -45.7252) -> (-301.2449, -47.7125) centre (-303.8596, 32.2447) ccw
  arc A300 (-303.3292, -31.8812) -> (-322.6379, -39.1123) centre (-285.1603, -109.7907) ccw
  line L213 (-149.3787, 125.3436) -> (-152.028, 152.028)
  line L214 (-219.5865, 129.6651) -> (-222.0865, 125.3349) construction
  line L215 (-204.766, 115.3349) -> (-239.407, 135.3349)
  arc A301 (-324.9588, 5.1732) -> (-305, 0) centre (-295.0744, 79.3819) ccw
  arc A302 (-304.582, 15.9625) -> (-324.7842, 11.8409) centre (-298.8246, -63.8301) ccw
  arc A303 (-302.3907, 39.8105) -> (-322.854, 37.2867) centre (-302.9114, -40.1878) ccw
  arc A304 (-323.5512, 30.6533) -> (-304.0598, 23.93) centre (-287.9366, 102.2884) ccw
  line L216 (-274.6528, 78.6819) -> (-279.3513, 80.392)
  arc A305 (-320.1488, 55.9443) -> (-301.2449, 47.7125) centre (-279.0235, 124.5644) ccw
  arc A306 (-298.335, 63.4131) -> (-318.9333, 62.5025) centre (-305.1308, -16.2978) ccw
  arc A307 (-314.7725, 80.8904) -> (-296.5728, 71.2008) centre (-268.3902, 146.0723) ccw
  arc A308 (-292.44, 86.6247) -> (-313.0462, 87.3331) centre (-305.4688, 7.6927) ccw
  line L217 (-279.3513, 80.392) -> (-265.6705, 117.9797)
  line L218 (-260.972, 116.2696) -> (-274.6528, 78.6819)
  line L219 (-279.3513, 80.392) -> (-260.972, 116.2696) construction
  line L220 (-265.6705, 117.9797) -> (-274.6528, 78.6819) construction
  arc A309 (-275.2885, 131.3059) -> (-295.5302, 135.2291) centre (-300.5046, 55.3839) ccw
  arc A310 (-298.2431, 129.1358) -> (-281.7833, 116.7184) centre (-242.2351, 186.2594) ccw
  arc A311 (-284.742, 109.3022) -> (-305.2291, 111.6252) centre (-303.9236, 31.6358) ccw
  arc A312 (-307.4556, 105.3378) -> (-290.0722, 94.2502) centre (-256.1021, 166.6797) ccw
  arc A313 (-287.1918, 152.1376) -> (-271.757, 138.4671) centre (-226.8746, 204.6908) ccw
  line L221 (-265.6705, 117.9797) -> (-260.972, 116.2696)
  line L222 (-270.1616, 98.3308) -> (-272.5109, 99.1858)
  arc A314 (-274.3699, 174.2014) -> (-260.0553, 159.3621) centre (-210.1154, 221.8601) ccw
  arc A315 (-251.3585, 172.7539) -> (-270.7372, 179.7953) centre (-288.1409, 101.7113) ccw
  arc A316 (-264.1377, 152.5) -> (-284.0092, 157.9993) centre (-295.2329, 78.7905) ccw
  line L223 (-210.6622, 176.7666) -> (-180.3122, 180.3122)
  arc A317 (-226.1226, 233.4386) -> (-215.6676, 215.6676) centre (-152.5177, 264.7806) ccw
  arc A318 (-221.2392, 209.9481) -> (-239.2778, 219.9344) centre (-268.6823, 145.5342) ccw
  arc A319 (-243.7409, 214.9776) -> (-231.9238, 198.0817) centre (-172.8219, 251.998) ccw
  arc A320 (-237.0295, 191.9427) -> (-255.7961, 200.4829) centre (-279.2725, 124.005) ccw
  arc A321 (-259.8565, 195.1912) -> (-246.7502, 179.2745) centre (-192.0607, 237.6617) ccw
  line L224 (-239.407, 135.3349) -> (-236.907, 139.6651)
  line L225 (0, 0) -> (-325, 0)
  line L226 (0, 0) -> (-229.8097, 229.8097)
  line L227 (0, 0) -> (-323.7633, -28.3256)
  line L228 (0, 0) -> (-248.9644, 208.906)
  line L229 (-202.266, 119.6651) -> (-204.766, 115.3349)
  line L230 (-238.157, 137.5) -> (-203.516, 117.5) construction
  line L231 (-236.907, 139.6651) -> (-204.766, 115.3349) construction
  line L232 (-236.907, 139.6651) -> (-202.266, 119.6651)
  line L233 (-239.407, 135.3349) -> (-202.266, 119.6651) construction
  line L234 (0, 0) -> (-324.8886, 8.5075) construction
  line L235 (0, 0) -> (-324.5546, 17.0092) construction
  line L236 (0, 0) -> (-300.3664, 52.9627)
  line L237 (0, 0) -> (-305.4001, 111.1565) construction
  line L238 (-226.7008, -155.6856) -> (-223.8329, -159.7814)
  line L239 (-223.8329, -159.7814) -> (-193.9347, -132.7426) construction
  line L240 (-193.9347, -132.7426) -> (-226.7008, -155.6856)
  line L241 (-225.2668, -157.7335) -> (-192.5007, -134.7905) construction
  line L242 (-226.7008, -155.6856) -> (-191.0668, -136.8383) construction
  line L243 (-223.8329, -159.7814) -> (-191.0668, -136.8383)
  line L244 (-191.0668, -136.8383) -> (-193.9347, -132.7426)
  line L245 (-125.3436, -149.3787) -> (-152.028, -152.028)
  line L246 (-176.7666, -210.6622) -> (-180.3122, -180.3122)
  arc A322 (-214.9776, -243.7409) -> (-198.0817, -231.9238) centre (-251.998, -172.8219) ccw
  arc A323 (-209.9481, -221.2392) -> (-219.9344, -239.2778) centre (-145.5342, -268.6823) ccw
  arc A324 (-195.1912, -259.8565) -> (-179.2745, -246.7502) centre (-237.6617, -192.0607) ccw
  arc A325 (-191.9427, -237.0295) -> (-200.4829, -255.7961) centre (-124.005, -279.2725) ccw
  line L247 (-194.258, -16.9954) -> (-215, 0)
  line L248 (-246.9581, -63.584) -> (-245.664, -68.4137) construction
  line L249 (-226.3455, -63.2373) -> (-264.9826, -73.5901)
  arc A326 (-233.4386, -226.1226) -> (-215.6676, -215.6676) centre (-264.7806, -152.5177) ccw
  arc A327 (-226.6592, -204.0848) -> (-238.0299, -221.2844) centre (-166.1662, -256.4356) ccw
  arc A328 (-241.9728, -185.6722) -> (-254.6579, -201.9266) centre (-185.7736, -242.6078) ccw
  arc A329 (-250.4604, -207.1101) -> (-231.9238, -198.0817) centre (-275.9308, -131.273) ccw
  line L250 (-249.8454, -138.5724) -> (-254.3769, -140.6855)
  arc A330 (-265.938, -186.8208) -> (-246.7502, -179.2745) centre (-285.3797, -109.2191) ccw
  arc A331 (-255.7945, -166.1149) -> (-269.7159, -181.3239) centre (-204.2358, -227.2843) ccw
  arc A332 (-279.776, -165.3796) -> (-260.0553, -159.3621) centre (-293.0692, -86.4918) ccw
  arc A333 (-268.0392, -145.5334) -> (-283.1109, -159.6033) centre (-221.4387, -210.5595) ccw
  line L251 (-254.3769, -140.6855) -> (-271.2816, -104.4331)
  line L252 (-266.7501, -102.32) -> (-249.8454, -138.5724)
  line L253 (-254.3769, -140.6855) -> (-266.7501, -102.32) construction
  line L254 (-271.2816, -104.4331) -> (-249.8454, -138.5724) construction
  arc A334 (-287.5057, -101.8111) -> (-304.5928, -113.35) centre (-251.6512, -173.3265) ccw
  arc A335 (-302.2025, -119.5769) -> (-281.7833, -116.7184) centre (-302.9913, -39.5808) ccw
  arc A336 (-278.6314, -124.0547) -> (-294.7605, -136.8987) centre (-237.2764, -192.5365) ccw
  arc A337 (-291.889, -142.9188) -> (-271.757, -138.4671) centre (-298.9518, -63.2312) ccw
  arc A338 (-310.6528, -95.4978) -> (-290.0722, -94.2502) centre (-305.1628, -15.6864) ccw
  line L255 (-271.2816, -104.4331) -> (-266.7501, -102.32)
  line L256 (-260.5635, -121.5028) -> (-262.8293, -122.5593)
  arc A339 (-317.1879, -70.8298) -> (-296.5728, -71.2008) centre (-305.4528, 8.3048) ccw
  arc A340 (-299.8927, -55.5818) -> (-318.5746, -64.3057) centre (-275.6672, -131.8257) ccw
  arc A341 (-294.6074, -78.9398) -> (-312.5472, -89.1025) centre (-264.4745, -153.0479) ccw
  line L257 (-273.9535, -23.9678) -> (-255, 0)
  arc A342 (-324.9588, 5.1732) -> (-305, 0) centre (-295.0744, 79.3819) ccw
  arc A343 (-304.8955, -7.984) -> (-324.712, -13.6779) centre (-292.8953, -87.0788) ccw
  arc A344 (-324.363, -20.3387) -> (-304.0598, -23.93) centre (-300.393, 55.9859) ccw
  arc A345 (-303.3292, -31.8812) -> (-322.6379, -39.1123) centre (-285.1603, -109.7907) ccw
  arc A346 (-321.7673, -45.7252) -> (-301.2449, -47.7125) centre (-303.8596, 32.2447) ccw
  line L258 (-264.9826, -73.5901) -> (-266.2766, -68.7604)
  line L259 (0, 0) -> (-229.8097, -229.8097)
  line L260 (0, 0) -> (-325, 0)
  line L261 (0, 0) -> (-208.906, -248.9644)
  line L262 (0, 0) -> (-323.7633, -28.3256)
  line L263 (-227.6396, -58.4077) -> (-226.3455, -63.2373)
  line L264 (-265.6296, -71.1752) -> (-226.9926, -60.8225) construction
  line L265 (-266.2766, -68.7604) -> (-226.3455, -63.2373) construction
  line L266 (-266.2766, -68.7604) -> (-227.6396, -58.4077)
  line L267 (-264.9826, -73.5901) -> (-227.6396, -58.4077) construction
  line L268 (0, 0) -> (-235.7467, -223.7152) construction
  line L269 (0, 0) -> (-241.5221, -217.4674) construction
  line L270 (0, 0) -> (-249.8414, -174.9408)
  line L271 (0, 0) -> (-294.55, -137.3509) construction
  point P0 (0, -165)
  point P1 (-116.6726, -116.6726)
  point P2 (-215.6676, -215.6676)
  point P3 (109.3022, 284.742)
  point P4 (111.6252, 305.2291)
  point P5 (105.3378, 307.4556)
  point P6 (94.2502, 290.0722)
  point P7 (86.6247, 292.44)
  point P8 (87.3331, 313.0462)
  point P9 (80.8904, 314.7725)
  point P10 (71.2008, 296.5728)
  point P11 (63.4131, 298.335)
  point P12 (62.5025, 318.9333)
  point P13 (55.9443, 320.1488)
  point P14 (47.7125, 301.2449)
  point P15 (39.8105, 302.3907)
  point P16 (37.2867, 322.854)
  point P17 (30.6533, 323.5512)
  point P18 (23.93, 304.0598)
  point P19 (-15.9625, -304.582)
  point P20 (-11.8409, -324.7842)
  point P21 (-37.3344, -211.7337)
  point P22 (-201.5254, -201.5254)
  point P23 (-183.1945, -218.3227)
  point P24 (-189.6223, -225.9831)
  point P25 (-208.5965, -208.5965)
  point P26 (0, -295)
  point P27 (-51.2262, -290.5183)
  point P28 (-49.4897, -280.6702)
  point P29 (0, -285)
  point P30 (0, -175)
  point P31 (-30.3884, -172.3414)
  point P32 (-28.6519, -162.4933)
  point P33 (-106.06, -126.3973)
  point P34 (-112.4878, -134.0578)
  point P35 (-123.7437, -123.7437)
  point P36 (-127.5, -220.8365)
  point P37 (15.2523, -174.3341)
  point P38 (-196.0502, -233.6436)
  point P39 (26.5825, -303.8394)
  point P40 (25.7109, -293.8774)
  point P41 (24.8394, -283.9155)
  point P42 (14.3807, -164.3721)
  point P43 (-219.9344, -239.2778)
  point P44 (-198.0817, -231.9238)
  point P45 (-200.4829, -255.7961)
  point P46 (-179.2745, -246.7502)
  point P47 (-172.7539, -251.3585)
  point P48 (-179.7953, -270.7372)
  point P49 (-174.2014, -274.3699)
  point P50 (-152.5, -264.1377)
  point P51 (-157.9993, -284.0092)
  point P52 (-138.4671, -271.757)
  point P53 (-135.2291, -295.5302)
  point P54 (-116.7184, -281.7833)
  point P55 (-109.3022, -284.742)
  point P56 (-111.6252, -305.2291)
  point P57 (-105.3378, -307.4556)
  point P58 (-94.2502, -290.0722)
  point P59 (-86.6247, -292.44)
  point P60 (-87.3331, -313.0462)
  point P61 (-80.8904, -314.7725)
  point P62 (-71.2008, -296.5728)
  point P63 (-63.4131, -298.335)
  point P64 (-62.5025, -318.9333)
  point P65 (-55.9443, -320.1488)
  point P66 (-47.7125, -301.2449)
  point P67 (-37.2867, -322.854)
  point P68 (-23.93, -304.0598)
  point P69 (242.2351, -186.2594)
  point P70 (65.9989, -246.3111)
  point P71 (210.1154, -221.8601)
  point P72 (63.8301, -298.8246)
  point P73 (-7.6927, -305.4688)
  point P74 (-15.9625, -304.582)
  point P75 (-23.93, -304.0598)
  point P76 (-31.6358, -303.9236)
  point P77 (16.2978, -305.1308)
  point P78 (40.1878, -302.9114)
  point P79 (305.1628, 15.6864)
  point P80 (220.8365, -127.5)
  point P81 (305.4528, -8.3048)
  point P82 (256.4356, -166.1662)
  point P83 (210.5595, -221.4387)
  point P84 (204.0848, -226.6592)
  point P85 (198.0817, -231.9238)
  point P86 (227.2843, -204.2358)
  point P87 (242.6078, -185.7736)
  point P88 (204.6908, 226.8746)
  point P89 (246.3111, 65.9989)
  point P90 (221.8601, 210.1154)
  point P91 (298.8246, 63.8301)
  point P92 (305.4688, -7.6927)
  point P93 (304.582, -15.9625)
  point P94 (304.0598, -23.93)
  point P95 (303.9236, -31.6358)
  point P96 (305.1308, 16.2978)
  point P97 (302.9114, 40.1878)
  point P98 (-15.6864, 305.1628)
  point P99 (-39.5808, 302.9913)
  point P100 (127.5, 220.8365)
  point P101 (8.3048, 305.4528)
  point P102 (166.1662, 256.4356)
  point P103 (221.4387, 210.5595)
  point P104 (226.6592, 204.0848)
  point P105 (231.9238, 198.0817)
  point P106 (237.2764, 192.5365)
  point P107 (204.2358, 227.2843)
  point P108 (185.7736, 242.6078)
  point P109 (-226.8746, 204.6908)
  point P110 (-242.2351, 186.2594)
  point P111 (-65.9989, 246.3111)
  point P112 (-210.1154, 221.8601)